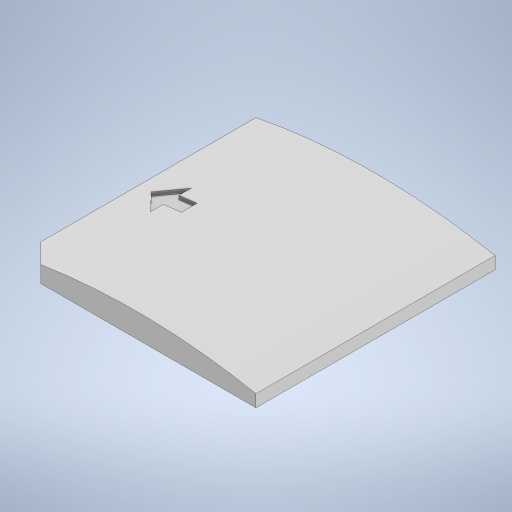
# Autodesk Inventor part: power_signal_socket_cap
Saved by Autodesk Inventor 2023 (Build 270158000, 158)
## iProperties
Created: 2023-09-07
Part Number: power_signal_socket_cap
Material: 一般
Document SubType Name: Modeling
Designer: 310611102
Density: 1 g/cm^3
Appearance: 預設
Author: 310611102
Autodesk Inventor part; units mm, degrees
ref_plane "YZ Plane" through (0, 0, 0) normal (1, 0, 0) x (0, 1, 0)
ref_plane "XY Plane" through (0, 0, 0) normal (0, 0, 1) x (1, 0, 0)
sketch "Sketch1" plane through (0, 0, 0) normal (0, 0, 1) x (1, 0, 0)
  line L0 (-25, 127.5735) -> (-25, 125)
  line L1 (-25, 125) -> (25, 125)
  line L2 (25, 125) -> (25, 127.5735)
  arc A0 (25, 127.5735) -> (-25, 127.5735) centre (0, 0) ccw
  point P0 (0, 130)
  dimension "d0" = 130
  dimension "d1" = 5
  dimension "d2" = 50
  constraints: 6 end point, 3 point on circle, 2 perpendicular, 1 centre point, 1 coincident, 1 vertical, 1 vertical alignment
  measures "d0" radius of A0
  measures "d1" distance from line of point (0, 130) L1
  measures "d2" distance of L0.end L1.end
extrude "Extrusion1" add sketch "Sketch1" along normal blind 50
chamfer "Chamfer1" distance 5 angle 45 1 edges at (-25, 126.2868, 50)
ref_plane "Work Plane1" through (0, 130, 0) normal (0, 1, 0) x (-1, 0, 0)
sketch "Sketch2" plane through (0, 130, 0) normal (0, 1, 0) x (-1, 0, 0)
  line L0 (20, 50) -> (-25, 50) construction
  line L1 (-25, 0) -> (-25, 50) construction
  line L2 (-25, 25) -> (31.0612, 25) construction
  line L3 (21.9246, 25) -> (17.7633, 29.2517)
  line L4 (17.7633, 29.2517) -> (17.7633, 26.6283)
  line L5 (17.7633, 26.6283) -> (13.964, 26.6283)
  line L6 (13.964, 26.6283) -> (13.964, 25)
  line L7 (21.9246, 25) -> (17.7633, 20.7483)
  line L8 (17.7633, 20.7483) -> (17.7633, 23.3717)
  line L9 (17.7633, 23.3717) -> (13.964, 23.3717)
  line L10 (13.964, 23.3717) -> (13.964, 25)
  point P0 (0, 0)
  constraints: 18 end point, 3 symmetric about line, 2 perpendicular, 2 point on line, 1 horizontal, 1 midpoint, 1 vertical
emboss "Emboss1" sketch "Sketch2" operation cut depth 0.8 direction (0, -1, 0)
sketch "Sketch3" plane through (-25, 125, 0) normal (0, -1, 0) x (1, 0, 0)
  line L0 (0, 0) -> (50, 0) projected
  line L1 (50, 0) -> (50, 50) construction
  line L2 (50, 25) -> (6.096, 25) construction
  circle A0 centre (18.5, 5) radius 3.5
  circle A1 centre (37.75, 5) radius 3.5
  circle A2 centre (18.5, 12.5) radius 2.75
  point P0 (25, 0)
  dimension "d20" = 7
  dimension "d21" = 7
  dimension "d22" = 20
  dimension "d23" = 20
  dimension "d24" = 12.25
  dimension "d25" = 19.25
  dimension "d26" = 5.5
  dimension "d27" = 12.5
  constraints: 3 centre point, 2 end point, 1 horizontal, 1 midpoint, 1 vertical alignment
  measures "d20" diameter of A0
  measures "d21" diameter of A1
  measures "d22" distance from line of L2 A0.centre
  measures "d23" distance from line of L2 A1.centre
  measures "d24" distance from line of L1 A1.centre
  measures "d25" distance of A1.centre A0.centre
  measures "d26" diameter of A2
  measures "d27" distance from line of L2 A2.centre
extrude "Extrusion2" cut sketch "Sketch3" against normal blind 2.5
ref_plane "Work Plane2" through (0, 0, 25) normal (0, 0, -1) x (-1, 0, 0)
mirror "Mirror1" about plane through (0, 0, 25) normal (0, 0, -1) of "Extrusion2"
body "Solid1"
